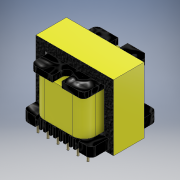
# Autodesk Inventor part: EI-31
Saved by Autodesk Inventor 2017.2 (Build 212223000, 223)
## iProperties
Part Number: EI-31
Material: Типовые
Document SubType Name: Modeling
Designer: Андрей
Density: 1 g/cm^3
Appearance: По умолчанию
Author: Андрей
Autodesk Inventor part; units mm, degrees
ref_plane "YZ Plane" through (0, 0, 0) normal (1, 0, 0) x (0, 1, 0)
ref_plane "XZ Plane" through (0, 0, 0) normal (0, 1, 0) x (-1, 0, 0)
ref_plane "XY Plane" through (0, 0, 0) normal (0, 0, 1) x (1, 0, 0)
sketch "Эскиз1" plane through (0, 0, 0) normal (0, 0, 1) x (1, 0, 0)
  line L0 (4, 0) -> (4, 6.5)
  line L1 (4, 6.5) -> (-4, 6.5)
  line L2 (-4, 6.5) -> (-4, -6.5)
  line L3 (-4, -6.5) -> (4, -6.5)
  line L4 (4, -6.5) -> (4, 0)
  point P0 (0, 0)
  dimension "d1" = 6.5
  dimension "d2" = 8
  dimension "d3" = 13
  dimension "d4" = 8
  constraints: 10 end point, 2 perpendicular, 1 point on line
  measures "d1" distance of L0.start L0.end
  measures "d2" distance of L0.end L1.end
  measures "d3" distance of L1.end L2.end
  measures "d4" distance of L2.end L3.end
sketch "Эскиз2" plane through (0, 0, 0) normal (0, 0, 1) x (1, 0, 0)
  line L0 (0, 14) -> (11.25, 14)
  line L1 (11.25, 14) -> (11.25, -14)
  line L2 (11.25, -14) -> (-11.25, -14)
  line L3 (-11.25, -14) -> (-11.25, 14)
  line L4 (-11.25, 14) -> (0, 14)
  line L5 (0, 0) -> (4, 0)
  line L6 (4, 0) -> (4, 6.5)
  line L7 (4, 6.5) -> (-4, 6.5)
  line L8 (-4, 6.5) -> (-4, -6.5)
  line L9 (-4, -6.5) -> (4, -6.5)
  line L10 (4, -6.5) -> (4, 0)
  dimension "d6" = 11.25
  dimension "d7" = 28
  dimension "d8" = 22.5
  dimension "d19" = 4
  dimension "d20" = 6.5
  dimension "d21" = 8
  dimension "d22" = 13
  dimension "d23" = 8
  constraints: 22 end point, 6 perpendicular, 2 collinear, 2 point on line, 1 horizontal
  measures "d6" distance of L0.start L0.end
  measures "d7" distance of L0.end L1.end
  measures "d8" distance of L1.end L2.end
  measures "d19" distance of L5.start L5.end
  measures "d20" distance of L5.end L6.end
  measures "d21" distance of L6.end L7.end
  measures "d22" distance of L7.end L8.end
  measures "d23" distance of L8.end L9.end
sketch "Эскиз3" plane through (0, 0, 0) normal (0, 0, 1) x (1, 0, 0)
  line L0 (0, 7.5) -> (5, 7.5)
  line L1 (5, 7.5) -> (5, -7.5)
  line L2 (5, -7.5) -> (-5, -7.5)
  line L3 (-5, -7.5) -> (-5, 7.5)
  line L4 (-5, 7.5) -> (0, 7.5)
  point P0 (0, 0)
  dimension "d10" = 5
  dimension "d12" = 15
  dimension "d13" = 10
  dimension "d14" = 15
  constraints: 10 end point, 2 perpendicular, 1 vertical
  measures "d10" distance of L0.start L0.end
  measures "d12" distance of L0.end L1.end
  measures "d13" distance of L1.end L2.end
  measures "d14" distance of L2.end L3.end
extrude "Выдавливание1" add sketch "Эскиз3" against normal blind 16
extrude "Выдавливание2" cut sketch "Эскиз1" against normal blind 16
extrude "Выдавливание3" add sketch "Эскиз2" along normal blind 2.5
fillet "Сопряжение1" radius 2 1 edges at (11.25, -14, 1.25)
sketch "Эскиз4" plane through (0, 0, 2.5) normal (0, 0, 1) x (1, 0, 0)
  line L0 (11.25, 14) -> (-11.25, 14) projected
  line L1 (0, 14) -> (0, 8)
  line L2 (-2, 10) -> (-2, 14)
  line L3 (2, 14) -> (-2, 14)
  arc A0 (-2, 10) -> (2, 10) centre (0, 10) ccw
  line L4 (2, 14) -> (2, 10)
  point P0 (0, 0)
  point P1 (9.25, 14)
  point P2 (-9.25, 14)
  constraints: 8 end point, 3 point on circle, 2 point on line, 2 vertical, 1 centre point, 1 collinear, 1 midpoint, 1 perpendicular
extrude "Выдавливание4" cut sketch "Эскиз4" against normal blind 2.5
chamfer "Фаска1" distance 2 angle 45 1 edges at (11.25, 14, 1.25)
fillet "Сопряжение3" radius 2 1 edges at (-11.25, -14, 1.25)
fillet "Сопряжение4" radius 2 1 edges at (-11.25, 14, 1.25)
sketch "Эскиз5" plane through (0, 0, -16) normal (0, 0, -1) x (-1, 0, 0)
  line L0 (4, 6.5) -> (-4, 6.5) projected
  line L1 (-4, 6.5) -> (4, 6.5)
  line L2 (4, -6.5) -> (4, 6.5) projected
  line L3 (4, 6.5) -> (4, -6.5)
  line L4 (-4, -6.5) -> (4, -6.5) projected
  line L5 (4, -6.5) -> (-4, -6.5)
  line L6 (-4, -6.5) -> (-4, 6.5)
  point P0 (0, 0)
  constraints: 8 end point, 3 collinear, 1 perpendicular
sketch "Эскиз6" plane through (0, 0, -16) normal (0, 0, -1) x (-1, 0, 0)
  line L0 (14.5, 0) -> (14.5, -14)
  line L1 (14.5, -14) -> (-14.5, -14)
  line L2 (-14.5, -14) -> (-14.5, 14)
  line L3 (-14.5, 14) -> (14.5, 14)
  line L4 (14.5, 14) -> (14.5, 0)
  point P0 (0, 0)
  dimension "d40" = 14
  dimension "d41" = 29
  dimension "d42" = 28
  dimension "d43" = 29
  constraints: 10 end point, 2 perpendicular, 1 point on line
  measures "d40" distance of L0.start L0.end
  measures "d41" distance of L0.end L1.end
  measures "d42" distance of L1.end L2.end
  measures "d43" distance of L2.end L3.end
extrude "Выдавливание5" add sketch "Эскиз6" along normal blind 4
extrude "Выдавливание6" cut sketch "Эскиз5" along normal blind 4
fillet "Сопряжение5" radius 2 1 edges at (-14.5, -14, -18)
fillet "Сопряжение6" radius 2 3 edges at (14.5, -14, -18) (14.5, 14, -18) (-14.5, 14, -18)
sketch "Эскиз7" plane through (0, 0, 2.5) normal (0, 0, 1) x (1, 0, 0)
  line L0 (-2, -10) -> (-2, -14)
  line L1 (-2, -14) -> (2, -14)
  line L2 (2, -14) -> (2, -10)
  arc A0 (2, -10) -> (-2, -10) centre (0, -10) ccw
  point P0 (0, 0)
  dimension "d53" = 4
  dimension "d54" = 4
  constraints: 6 end point, 2 point on circle, 1 centre point, 1 perpendicular, 1 point on line, 1 tangent
  measures "d53" distance of L0.end L1.end
  measures "d54" distance of L1.end L2.end
extrude "Выдавливание7" cut sketch "Эскиз7" against normal blind 2.5
sketch "Эскиз8" plane through (0, 0, -20) normal (0, 0, -1) x (-1, 0, 0)
  circle A0 centre (-10.625, -11.46) radius 0.4
  point P0 (0, 0)
  constraints: 1 centre point
extrude "Выдавливание8" add sketch "Эскиз8" along normal blind 4
chamfer "Фаска2" distance 0.1 angle 45 1 edges at (11.025, -11.46, -24)
sketch "Эскиз9" plane through (0, 0, -20) normal (0, 0, -1) x (-1, 0, 0)
  circle A0 centre (-10.625, -11.46) radius 0.4 projected
  circle A1 centre (-6.375, -11.46) radius 0.4
  point P0 (0, 0)
  constraints: 1 centre point
extrude "Выдавливание9" add sketch "Эскиз9" along normal blind 4 contours A1
chamfer "Фаска3" distance 0.1 angle 45 1 edges at (6.775, -11.46, -24)
sketch "Эскиз10" plane through (0, 0, -20) normal (0, 0, -1) x (-1, 0, 0)
  circle A0 centre (-6.375, -11.46) radius 0.4 projected
  circle A1 centre (-2.125, -11.46) radius 0.4
  point P0 (0, 0)
  constraints: 1 centre point
extrude "Выдавливание10" add sketch "Эскиз10" along normal blind 4 contours A1
chamfer "Фаска4" distance 0.1 angle 45 1 edges at (2.525, -11.46, -24)
sketch "Эскиз11" plane through (0, 0, -20) normal (0, 0, -1) x (-1, 0, 0)
  circle A0 centre (-2.125, -11.46) radius 0.4 projected
  circle A1 centre (2.125, -11.46) radius 0.4
  point P0 (0, 0)
  constraints: 1 centre point
extrude "Выдавливание11" add sketch "Эскиз11" along normal blind 4 contours A1
chamfer "Фаска5" distance 0.1 angle 45 1 edges at (-1.725, -11.46, -24)
sketch "Эскиз12" plane through (0, 0, -20) normal (0, 0, -1) x (-1, 0, 0)
  circle A0 centre (2.125, -11.46) radius 0.3 projected
  circle A1 centre (6.375, -11.46) radius 0.4
  point P0 (0, 0)
  constraints: 1 centre point
extrude "Выдавливание12" add sketch "Эскиз12" along normal blind 4 contours A1
chamfer "Фаска6" distance 0.1 angle 45 1 edges at (-5.975, -11.46, -24)
sketch "Эскиз13" plane through (0, 0, -20) normal (0, 0, -1) x (-1, 0, 0)
  circle A0 centre (6.375, -11.46) radius 0.3 projected
  circle A1 centre (10.625, -11.46) radius 0.4
  point P0 (0, 0)
  constraints: 1 centre point
extrude "Выдавливание13" add sketch "Эскиз13" along normal blind 4 contours A1
chamfer "Фаска7" distance 0.1 angle 45 1 edges at (-10.225, -11.46, -24)
sketch "Эскиз14" plane through (0, 0, -20) normal (0, 0, -1) x (-1, 0, 0)
  circle A0 centre (-6.375, -11.46) radius 0.4 projected
  line L0 (-12.5, -14) -> (12.5, -14) projected
  line L1 (-5, -10.25) -> (-5, -14)
  line L2 (-3.5, -10.25) -> (-3.5, -14)
  arc A1 (-3.5, -10.25) -> (-5, -10.25) centre (-4.25, -10.25) ccw
  point P0 (0, 0)
  constraints: 4 end point, 2 point on circle, 2 point on line, 1 centre point
extrude "Выдавливание14" cut sketch "Эскиз14" against normal blind 4 contours L1 A1 L2 L0
sketch "Эскиз15" plane through (0, 0, -20) normal (0, 0, -1) x (-1, 0, 0)
  line L0 (-0.75, -10.25) -> (-0.75, -14)
  line L1 (-3.5, -14) -> (12.5, -14) projected
  line L2 (0.75, -10.25) -> (0.75, -14)
  arc A0 (0.75, -10.25) -> (-0.75, -10.25) centre (0, -10.25) ccw
  point P0 (0, 0)
  constraints: 4 end point, 2 point on circle, 2 point on line, 1 centre point
extrude "Выдавливание15" cut sketch "Эскиз15" against normal blind 4
sketch "Эскиз16" plane through (0, 0, -20) normal (0, 0, -1) x (-1, 0, 0)
  circle A0 centre (2.125, -11.46) radius 0.3 projected
  line L0 (3.5, -9.75) -> (3.5, -14)
  line L1 (0.75, -14) -> (12.5, -14) projected
  line L2 (5, -9.75) -> (5, -14)
  arc A1 (5, -9.75) -> (3.5, -9.75) centre (4.25, -9.75) ccw
  point P0 (0, 0)
  constraints: 4 end point, 2 point on circle, 2 point on line, 1 centre point
extrude "Выдавливание16" cut sketch "Эскиз16" against normal blind 4 contours A1 L2 L1 L0
sketch "Эскиз17" plane through (0, 0, -20) normal (0, 0, -1) x (-1, 0, 0)
  circle A0 centre (-10.625, -11.46) radius 0.3 projected
  line L0 (-9.25, -12.2451) -> (-9.25, -14)
  line L1 (-7.75, -12.2451) -> (-7.75, -14)
  line L2 (-7.75, -14) -> (-9.25, -14)
  line L3 (-5, -14) -> (-12.5, -14) projected
  arc A1 (-7.75, -12.2451) -> (-9.25, -12.2451) centre (-8.5, -12.2451) ccw
  point P0 (0, 0)
  constraints: 6 end point, 2 point on circle, 1 centre point, 1 collinear
extrude "Выдавливание17" cut sketch "Эскиз17" against normal blind 4 contours A1 L1 L2 L0
sketch "Эскиз19" plane through (0, 0, -20) normal (0, 0, -1) x (-1, 0, 0)
  line L0 (-2, -14) -> (-9.25, -14)
  line L1 (-5, -14) -> (-6.375, -14)
  line L2 (-6.375, -14) -> (-5.375, -14)
  line L3 (-6.875, -13.5) -> (-6.875, -14)
  line L4 (-2, -14) -> (-9.25, -14) projected
  line L5 (-5.875, -13.5) -> (-5.875, -14)
  arc A0 (-5.875, -13.5) -> (-6.875, -13.5) centre (-6.375, -13.5) ccw
  point P0 (0, 0)
  constraints: 10 end point, 5 point on line, 2 point on circle, 1 centre point
extrude "Выдавливание19" cut sketch "Эскиз19" against normal blind 4
sketch "Эскиз20" plane through (0, 0, -20) normal (0, 0, -1) x (-1, 0, 0)
  circle A0 centre (-2.125, -11.46) radius 0.3 projected
  line L0 (-2.625, -14) -> (-2.625, -13.5)
  line L1 (-1.625, -13.5) -> (-1.625, -14)
  arc A1 (-1.625, -13.5) -> (-2.625, -13.5) centre (-2.125, -13.5) ccw
  line L2 (-1.625, -14) -> (-2.625, -14)
  line L3 (-3.5, -14) -> (-0.75, -14) projected
  point P0 (0, 0)
  constraints: 6 end point, 2 point on circle, 1 centre point, 1 collinear
extrude "Выдавливание20" cut sketch "Эскиз20" against normal blind 4 contours L0 A1 L1 L2
sketch "Эскиз21" plane through (0, 0, -20) normal (0, 0, -1) x (-1, 0, 0)
  circle A0 centre (2.125, -11.46) radius 0.3 projected
  line L0 (3.5, -14) -> (0.75, -14) projected
  line L1 (1.625, -14) -> (1.625, -13.5)
  line L2 (2.625, -13.5) -> (2.625, -14)
  line L3 (2.625, -14) -> (1.625, -14)
  arc A1 (2.625, -13.5) -> (1.625, -13.5) centre (2.125, -13.5) ccw
  point P0 (0, 0)
  constraints: 6 end point, 2 point on circle, 2 point on line, 1 centre point, 1 perpendicular
extrude "Выдавливание21" cut sketch "Эскиз21" against normal blind 4 contours L0 L1 A1 L2
sketch "Эскиз22" plane through (0, 0, -20) normal (0, 0, -1) x (-1, 0, 0)
  line L0 (5.875, -13.5) -> (5.875, -14)
  line L1 (5, -14) -> (-9.25, -14) projected
  line L2 (6.875, -13.5) -> (6.875, -14)
  arc A0 (6.875, -13.5) -> (5.875, -13.5) centre (6.375, -13.5) ccw
  line L3 (6.875, -14) -> (5.875, -14)
  line L4 (2, -14) -> (9.25, -14) projected
  point P0 (0, 0)
  point P1 (7.25, -14)
  constraints: 6 end point, 2 point on circle, 2 point on line, 1 centre point, 1 collinear
extrude "Выдавливание22" cut sketch "Эскиз22" against normal blind 4
sketch "Эскиз23" plane through (0, 0, -20) normal (0, 0, -1) x (-1, 0, 0)
  line L0 (9.25, -12.25) -> (9.25, -14)
  line L1 (7.75, -12.25) -> (7.75, -14)
  arc A0 (9.25, -12.25) -> (7.75, -12.25) centre (8.5, -12.25) ccw
  line L2 (9.25, -14) -> (7.75, -14)
  line L3 (12.5, -14) -> (6.875, -14) projected
  point P0 (0, 0)
  constraints: 6 end point, 2 point on circle, 1 centre point, 1 collinear
extrude "Выдавливание23" cut sketch "Эскиз23" against normal blind 4
sketch "Эскиз24" plane through (0, 0, -20) normal (0, 0, -1) x (-1, 0, 0)
  arc A0 (9.25, -12.25) -> (7.75, -12.25) centre (8.5, -12.25) ccw projected
  line L0 (8.5, -12.25) -> (8.5, 17)
  arc A1 (5, -9.75) -> (3.5, -9.75) centre (4.25, -9.75) ccw projected
  line L1 (4.25, -9.75) -> (4.25, 26)
  line L2 (-12.5, 14) -> (12.5, 14) projected
  line L3 (8.5, 14) -> (8.5, 11.5)
  line L4 (9.25, 12.25) -> (9.25, 14)
  line L5 (7.75, 12.25) -> (7.75, 14)
  arc A2 (7.75, 12.25) -> (9.25, 12.25) centre (8.5, 12.25) ccw
  line L6 (7.75, 14) -> (9.25, 14)
  point P0 (0, 0)
  constraints: 12 end point, 5 point on line, 3 point on circle, 2 vertical, 1 centre point, 1 collinear
extrude "Выдавливание24" cut sketch "Эскиз24" against normal blind 4
sketch "Эскиз25" plane through (0, 0, -20) normal (0, 0, -1) x (-1, 0, 0)
  arc A0 (-7.75, -12.2451) -> (-9.25, -12.2451) centre (-8.5, -12.2451) ccw projected
  line L0 (-7.75, 12.25) -> (-7.75, 14)
  line L1 (-9.25, 12.25) -> (-9.25, 14)
  line L2 (-9.25, 14) -> (-7.75, 14)
  arc A1 (-9.25, 12.25) -> (-7.75, 12.25) centre (-8.5, 12.25) ccw
  point P0 (0, 0)
  constraints: 6 end point, 2 point on circle, 1 centre point
extrude "Выдавливание25" cut sketch "Эскиз25" against normal blind 4
sketch "Эскиз26" plane through (0, 0, -20) normal (0, 0, -1) x (-1, 0, 0)
  line L0 (-6.875, 14) -> (-6.875, 13.5)
  line L1 (-5.875, 13.5) -> (-5.875, 14)
  line L2 (-5.875, 14) -> (-6.875, 14)
  line L3 (-5.875, 14) -> (-6.875, 14)
  line L4 (-7.75, 14) -> (7.75, 14) projected
  arc A0 (-6.875, 13.5) -> (-5.875, 13.5) centre (-6.375, 13.5) ccw
  point P0 (0, 0)
  constraints: 8 end point, 2 point on circle, 1 centre point, 1 collinear
extrude "Выдавливание26" cut sketch "Эскиз26" against normal blind 4
sketch "Эскиз27" plane through (0, 0, -20) normal (0, 0, -1) x (-1, 0, 0)
  line L0 (7.75, 12.25) -> (7.75, 14) projected
  line L1 (7.75, 14) -> (-5.875, 14) projected
  line L2 (6.875, 14) -> (6.875, 13.5)
  line L3 (5.875, 13.5) -> (5.875, 14)
  arc A0 (5.875, 13.5) -> (6.875, 13.5) centre (6.375, 13.5) ccw
  line L4 (6.875, 14) -> (5.875, 14)
  point P0 (0, 0)
  constraints: 6 end point, 2 point on circle, 2 point on line, 1 centre point, 1 collinear
extrude "Выдавливание27" cut sketch "Эскиз27" against normal blind 4
sketch "Эскиз28" plane through (0, 0, -20) normal (0, 0, -1) x (-1, 0, 0)
  line L0 (5, 14) -> (5, 9.75)
  line L1 (3.5, 9.75) -> (3.5, 14)
  line L2 (-5.875, 14) -> (5.875, 14) projected
  arc A0 (3.5, 9.75) -> (5, 9.75) centre (4.25, 9.75) ccw
  line L3 (3.5, 14) -> (5, 14)
  point P0 (0, 0)
  constraints: 6 end point, 2 point on circle, 1 centre point, 1 collinear
extrude "Выдавливание28" cut sketch "Эскиз28" against normal blind 4
sketch "Эскиз29" plane through (0, 0, -20) normal (0, 0, -1) x (-1, 0, 0)
  line L0 (3.5, 14) -> (-5.875, 14) projected
  line L1 (2.625, 14) -> (2.625, 13.5)
  line L2 (1.625, 13.5) -> (1.625, 14)
  line L3 (1.625, 14) -> (2.625, 14)
  arc A0 (1.625, 13.5) -> (2.625, 13.5) centre (2.125, 13.5) ccw
  point P0 (0, 0)
  constraints: 6 end point, 2 point on circle, 2 point on line, 1 centre point
extrude "Выдавливание29" cut sketch "Эскиз29" against normal blind 4
sketch "Эскиз30" plane through (0, 0, -20) normal (0, 0, -1) x (-1, 0, 0)
  line L0 (1.625, 14) -> (1.625, 13.5) projected
  line L1 (-5.875, 14) -> (1.625, 14) projected
  line L2 (0.75, 14) -> (0.75, 9.75)
  line L3 (-0.75, 9.75) -> (-0.75, 14)
  arc A0 (-0.75, 9.75) -> (0.75, 9.75) centre (0, 9.75) ccw
  line L4 (-0.75, 14) -> (0.75, 14)
  point P0 (0, 0)
  constraints: 6 end point, 2 point on circle, 1 centre point, 1 collinear, 1 point on line
extrude "Выдавливание30" cut sketch "Эскиз30" against normal blind 4
sketch "Эскиз31" plane through (0, 0, -20) normal (0, 0, -1) x (-1, 0, 0)
  line L0 (-0.75, 14) -> (-5.875, 14) projected
  line L1 (-0.75, 14) -> (-1.625, 14)
  line L2 (-1.625, 14) -> (-1.625, 13.5)
  line L3 (-2.625, 13.5) -> (-2.625, 14)
  line L4 (-2.625, 14) -> (-1.625, 14)
  arc A0 (-2.625, 13.5) -> (-1.625, 13.5) centre (-2.125, 13.5) ccw
  point P0 (0, 0)
  constraints: 8 end point, 2 point on circle, 2 point on line, 1 centre point, 1 perpendicular
extrude "Выдавливание31" cut sketch "Эскиз31" against normal blind 4
sketch "Эскиз32" plane through (0, 0, -20) normal (0, 0, -1) x (-1, 0, 0)
  line L0 (-2.625, 14) -> (-3.5, 14)
  line L1 (-3.5, 14) -> (-3.5, 9.75)
  line L2 (-5, 9.75) -> (-5, 14)
  arc A0 (-5, 9.75) -> (-3.5, 9.75) centre (-4.25, 9.75) ccw
  line L3 (-5, 14) -> (-3.5, 14)
  line L4 (-5.875, 14) -> (-2.625, 14) projected
  point P0 (0, 0)
  constraints: 8 end point, 2 point on circle, 1 centre point, 1 collinear, 1 perpendicular
extrude "Выдавливание32" cut sketch "Эскиз32" against normal blind 4
sketch "Эскиз33" plane through (0, 0, -20) normal (0, 0, -1) x (-1, 0, 0)
  circle A0 centre (-6.375, -11.46) radius 0.3 projected
  line L0 (-2, 14) -> (-9.25, 14) projected
  circle A1 centre (-6.375, 11.46) radius 0.4
  point P0 (0, 0)
  constraints: 1 centre point
extrude "Выдавливание33" add sketch "Эскиз33" along normal blind 4 contours A1
chamfer "Фаска8" distance 0.1 angle 45 1 edges at (6.775, 11.46, -24)
sketch "Эскиз34" plane through (0, 0, -20) normal (0, 0, -1) x (-1, 0, 0)
  circle A0 centre (-2.125, -11.46) radius 0.4 projected
  circle A1 centre (-2.125, 11.46) radius 0.4
  point P0 (0, 0)
  constraints: 1 centre point
extrude "Выдавливание34" add sketch "Эскиз34" along normal blind 4 contours A1
chamfer "Фаска9" distance 0.1 angle 45 1 edges at (2.525, 11.46, -24)
sketch "Эскиз35" plane through (0, 0, -20) normal (0, 0, -1) x (-1, 0, 0)
  circle A0 centre (2.125, -11.46) radius 0.4 projected
  circle A1 centre (2.125, 11.46) radius 0.4
  point P0 (0, 0)
  constraints: 1 centre point
extrude "Выдавливание35" add sketch "Эскиз35" along normal blind 4 contours A1
chamfer "Фаска10" distance 0.1 angle 45 1 edges at (-1.725, 11.46, -24)
sketch "Эскиз36" plane through (0, 0, -16) normal (0, 0, 1) x (1, 0, 0)
  line L0 (-5, -7.5) -> (-5, 7.5) projected
  line L1 (-5, 7.5) -> (5, 7.5) projected
  line L2 (-5, 7.5) -> (5, 7.5)
  line L3 (5, -7.5) -> (-5, -7.5) projected
  line L4 (5, 7.5) -> (5, -7.5)
  line L5 (5, -7.5) -> (-5, -7.5)
  line L6 (-5, -7.5) -> (-5, 7.5)
  line L7 (-4, 6.5) -> (-4, -6.5) projected
  line L8 (-3.5, 9.75) -> (-3.5, 14) projected
  line L9 (4, -6.5) -> (4, 6.5) projected
  line L10 (-4, -6.5) -> (4, -6.5) projected
  line L11 (-11, -6.5) -> (-11, 6.5)
  line L12 (-11, 6.5) -> (-11, 13.5)
  line L13 (-11, -6.5) -> (-11, -13.5)
  line L14 (11, 13.5) -> (11, -13.5)
  line L15 (-11, -13.5) -> (-11, 13.5)
  line L16 (-11, -13.5) -> (11, -13.5)
  line L17 (-11, 13.5) -> (11, 13.5)
  point P0 (0, 0)
  constraints: 22 end point, 2 collinear, 2 horizontal, 2 perpendicular, 2 vertical, 1 point on line
extrude "Выдавливание36" add sketch "Эскиз36" along normal blind 16
fillet "Сопряжение7" radius 5 1 edges at (11, -13.5, -8)
fillet "Сопряжение8" radius 5 3 edges at (11, 13.5, -8) (-11, -13.5, -8) (-11, 13.5, -8)
sketch "Эскиз38" plane through (0, 0, 2.5) normal (0, 0, 1) x (1, 0, 0)
  line L0 (-4, 6.5) -> (4, 6.5) projected
  line L1 (16.5, 6.5) -> (16.5, -6.5)
  line L2 (16.5, -6.5) -> (-16.5, -6.5)
  line L3 (-16.5, -6.5) -> (-16.5, 6.5)
  line L4 (-16.5, 6.5) -> (16.5, 6.5)
  point P0 (0, 0)
  dimension "d326" = 13
  dimension "d327" = 33
  dimension "d328" = 13
  constraints: 8 end point, 2 perpendicular
  measures "d326" distance of L1.start L1.end
  measures "d327" distance of L1.end L2.end
  measures "d328" distance of L2.end L3.end
extrude "Выдавливание37" add sketch "Эскиз38" along normal blind 4
sketch "Эскиз39" plane through (0, 0, 2.5) normal (0, 0, -1) x (-1, 0, 0)
  point P0 (0, 0)
sketch "Эскиз40" plane through (0, 0, -20) normal (0, 0, -1) x (-1, 0, 0)
  line L0 (-16.5, 6.5) -> (-16.5, -6.5) projected
  line L1 (-16.5, -6.5) -> (-12, -6.5)
  line L2 (16.5, -6.5) -> (-16.5, -6.5) projected
  line L3 (-12, -6.5) -> (-12, 6.5)
  line L4 (-12, 6.5) -> (-16.5, 6.5)
  line L5 (-16.5, 6.5) -> (-16.5, -6.5)
  point P0 (0, 0)
  dimension "d331" = 4.5
  dimension "d332" = 13
  constraints: 8 end point, 3 perpendicular, 1 point on line
  measures "d331" distance of L0.end L1.end
  measures "d332" distance of L1.end L3.end
extrude "Выдавливание38" cut sketch "Эскиз40" against normal blind 4
sketch "Эскиз41" plane through (0, 0, -20) normal (0, 0, -1) x (-1, 0, 0)
  line L0 (16.5, -6.5) -> (16.5, 6.5) projected
  line L1 (16.5, -6.5) -> (12, -6.5)
  line L2 (11.25, -6.5) -> (16.5, -6.5) projected
  line L3 (11.25, -6.5) -> (11.25, 6.5)
  line L4 (16.5, 6.5) -> (11.25, 6.5) projected
  line L5 (11.25, 6.5) -> (16.5, 6.5)
  line L6 (16.5, 6.5) -> (16.5, -6.5)
  point P0 (0, 0)
  dimension "d335" = 4.5
  constraints: 8 end point, 1 collinear, 1 perpendicular, 1 point on line, 1 vertical
  measures "d335" distance of L0.start L1.end
extrude "Выдавливание39" cut sketch "Эскиз41" against normal blind 4
sketch "Эскиз42" plane through (0, 0, -20) normal (0, 0, -1) x (-1, 0, 0)
  line L0 (-12, 6.5) -> (-12, -6.5) projected
  line L1 (-12, -6.5) -> (-12, 6.5)
  line L2 (14.5, 6.5) -> (11.25, 6.5) projected
  line L3 (-12, 6.5) -> (11.25, 6.5)
  line L4 (11.25, 6.5) -> (11.25, -6.5)
  line L5 (11, -8.5) -> (11, 8.5) projected
  line L6 (11.25, -6.5) -> (-12, -6.5)
  point P0 (0, 0)
  constraints: 8 end point, 2 collinear, 1 parallel, 1 perpendicular
extrude "Выдавливание40" cut sketch "Эскиз42" against normal blind 3
sketch "Эскиз43" plane through (0, 0, 2.5) normal (0, 0, -1) x (-1, 0, 0)
  line L0 (-16.5, 6.5) -> (-16.5, -6.5) projected
  line L1 (-16.5, -6.5) -> (-16.5, 6.5)
  line L2 (-16.5, 6.5) -> (-12.5, 6.5)
  line L3 (-12.5, 6.5) -> (-12.5, -6.5)
  line L4 (-16.5, -6.5) -> (-11.25, -6.5) projected
  line L5 (-12.5, -6.5) -> (-16.5, -6.5)
  point P0 (0, 0)
  dimension "d340" = 4
  constraints: 8 end point, 2 perpendicular, 1 collinear, 1 vertical
  measures "d340" distance of L0.start L2.end
extrude "Выдавливание41" add sketch "Эскиз43" along normal blind 20
sketch "Эскиз44" plane through (0, 0, 2.5) normal (0, 0, -1) x (-1, 0, 0)
  line L0 (16.5, -6.5) -> (16.5, 6.5) projected
  line L1 (16.5, 6.5) -> (16.5, -6.5)
  line L2 (16.5, -6.5) -> (12.5, -6.5)
  line L3 (11.25, -6.5) -> (14.5, -6.5) projected
  line L4 (12.5, -6.5) -> (12.5, 6.5)
  line L5 (14.5, 6.5) -> (11.25, 6.5) projected
  line L6 (16.5, 6.5) -> (11.25, 6.5) projected
  line L7 (12.5, 6.5) -> (16.5, 6.5)
  point P0 (0, 0)
  dimension "d343" = 4
  constraints: 8 end point, 2 point on line, 1 collinear, 1 horizontal, 1 perpendicular
  measures "d343" distance of L0.start L2.end
extrude "Выдавливание42" add sketch "Эскиз44" along normal blind 20
sketch "Эскиз45" plane through (0, 0, -17.5) normal (0, 0, -1) x (-1, 0, 0)
  line L0 (-16.5, -6.5) -> (-16.5, 6.5) projected
  line L1 (16.5, 6.5) -> (14.5, 6.5) projected
  line L2 (-16.5, 6.5) -> (16.5, 6.5)
  line L3 (14.5, -6.5) -> (16.5, -6.5) projected
  line L4 (16.5, 6.5) -> (16.5, -6.5)
  line L5 (16.5, -6.5) -> (-16.5, -6.5)
  line L6 (-16.5, -6.5) -> (-16.5, 6.5)
  point P0 (0, 0)
  constraints: 8 end point, 3 perpendicular, 1 collinear
extrude "Выдавливание43" add sketch "Эскиз45" along normal blind 4
